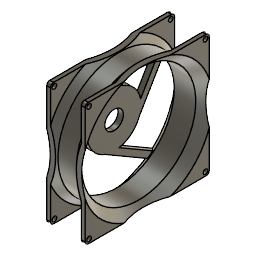
cooling_fan_pro (Autodesk Fusion 360 archive; units mm, degrees)
design "cooling fan case"
part number: 2026-04-21-22-51-45-922
Autodesk Fusion 360 part; units mm, degrees
sketch "Sketch1" plane through (0, 0, 0) normal (0, 1, 0) x (1, 0, 0)
  line L0 (0, 0) -> (7, 0)
  line L1 (7, 0) -> (12, 0) construction
  line L2 (12.5, -5.5) -> (12.5, -19.5)
  line L3 (7, 0) -> (12.5, -5.5)
  line L4 (0, -2.5) -> (5.9645, -2.5)
  line L5 (5.9645, -2.5) -> (10, -6.5355)
  line L6 (10, -6.5355) -> (10, -19.5)
  line L7 (10, -19.5) -> (12.5, -19.5)
  line L8 (0, 1) -> (0, -23) construction
  line L9 (-5.9645, -2.5) -> (-10, -6.5355)
  line L10 (-7, 0) -> (-12, 0) construction
  line L11 (0, -2.5) -> (-5.9645, -2.5)
  line L12 (0, 0) -> (-7, 0)
  line L13 (-12.5, -5.5) -> (-12.5, -19.5)
  line L14 (-10, -19.5) -> (-12.5, -19.5)
  line L15 (-7, 0) -> (-12.5, -5.5)
  line L16 (-10, -6.5355) -> (-10, -19.5)
  line L17 (0, 0) -> (0, 37) construction
  line L18 (0, 37) -> (31.2088, 37)
  dimension "d1" = 7
  dimension "d4" = 14
  dimension "d7" = 5.5
  dimension "d8" = 5.5
  dimension "d9" = 2.5
  dimension "d10" = 37
  constraint coincident L0.start L12.start
  constraint horizontal L0
  constraint horizontal L1
  constraint vertical L2
  constraint perpendicular L2 L7
  constraint perpendicular L0 L8
  constraint symmetric L0.start L8 L12.start
  constraint symmetric L0.end L8 L10.start
  constraint symmetric L2.start L8 L13.start
  constraint symmetric L1.end L8 L10.end
  constraint symmetric L2.end L8 L13.end
  constraint symmetric L4.start L8 L11.start
  constraint symmetric L4.end L8 L9.start
  constraint symmetric L5.end L8 L9.end
  constraint symmetric L6.end L8 L14.start
  constraint perpendicular L10 L17
  constraint perpendicular L17 L18
  measures "d1" distance of L0.start L0.end
  measures "d4" distance of L2.start L2.end
  measures "d7" vertical distance of L0.end L2.start
  measures "d8" horizontal distance of L0.end L2.start
  measures "d10" distance of L0.start L17.end
revolve "Revolve1" add sketch "Sketch1" angle 360 about axis through (0, 0, -37) along (1, 0, 0)
sketch "Sketch2" plane through (-12.5, 0, 0) normal (-1, 0, 0) x (0, -1, 0)
  circle A0 centre (0, -37) radius 56.5
  circle A1 centre (0, -37) radius 42.5
  circle A2 centre (0, -37) radius 56.5
  line L0 (40.2807, 2.75) -> (-40.2807, 2.75)
  line L1 (-40.2807, 2.75) -> (-40.2807, -76.75)
  line L2 (-40.2807, -76.75) -> (40.2807, -76.75)
  line L3 (40.2807, -76.75) -> (40.2807, 2.75)
  line L4 (40.2807, 2.75) -> (-40.2807, -76.75) construction
  line L5 (-40.2807, 2.75) -> (40.2807, -76.75) construction
  line L6 (72, 35) -> (-72, 35)
  line L7 (-72, 35) -> (-72, -109)
  line L8 (-72, -109) -> (72, -109)
  line L9 (72, -109) -> (72, 35)
  line L10 (72, 35) -> (-72, -109) construction
  line L11 (-72, 35) -> (72, -109) construction
  point P0 (0, -37)
  point P1 (0, -37)
  dimension "d12" = 79.5
  dimension "d13" = 144
  dimension "d14" = 144
  constraint horizontal L0
  constraint perpendicular L0 L1
  constraint parallel L0 L2
  constraint parallel L1 L3
  constraint coincident L4 P1
  constraint coincident L5 P1
  constraint coincident P1 P0
  constraint horizontal L6
  constraint perpendicular L6 L7
  constraint parallel L6 L8
  constraint parallel L7 L9
  constraint coincident L10 P1
  constraint coincident L11 P1
  measures "d12" distance of L0.end L1.end
  measures "d13" distance of L7.end L8.end
  measures "d14" distance of L6.end L7.end
extrude "Extrude1" cut sketch "Sketch2" along normal mid plane 220 contours A0 A1 A2 L3 | A0 A1 A2 L0 | A1 L3 | A0 A1 A2 L2 | A1 L0 | A1 L2 | A0 A1 A2 L1 | A1 L1 | L6 L7 L8 L9
sketch "Sketch3" plane through (-12.5, 0, 0) normal (-1, 0, 0) x (0, -1, 0)
  line L0 (40.1521, 2.75) -> (15.0395, 2.75)
  arc A0 (40.2807, -23.4459) -> (15.0395, 2.75) centre (0, -37) ccw
  line L1 (40.2807, -23.4459) -> (40.2807, 2.6196)
  arc A1 (40.2807, 2.6196) -> (40.1521, 2.75) centre (0, -37) ccw
  circle A2 centre (37.7807, 0.25) radius 1.5
  dimension "d17" = 3
  dimension "d18" = 2.5
  dimension "d19" = 2.5
  measures "d17" diameter of A2
  measures "d18" distance of L0 A2.centre
  measures "d19" distance of L1 A2.centre
extrude "Extrude2" cut sketch "Sketch3" against normal blind 95 contours A2
sketch "Sketch4" plane through (-12.5, 0, 0) normal (-1, 0, 0) x (0, -1, 0)
  circle A0 centre (37.7807, 0.25) radius 1.5
  line L0 (40.1521, 2.75) -> (15.0395, 2.75)
  arc A1 (40.2807, -23.4459) -> (15.0395, 2.75) centre (0, -37) ccw
  line L1 (40.2807, -23.4459) -> (40.2807, 2.6196)
  arc A2 (40.2807, 2.6196) -> (40.1521, 2.75) centre (0, -37) ccw
  circle A3 centre (-37.7807, 0.25) radius 1.5
  line L2 (-15.0395, 2.75) -> (-40.1521, 2.75)
  line L3 (-40.2807, 2.6196) -> (-40.2807, -23.4459)
  dimension "d22" = 3
  dimension "d23" = 2.5
  dimension "d24" = 2.5
  measures "d22" diameter of A3
  measures "d23" distance of A3.centre L2
  measures "d24" distance of A3.centre L3
extrude "Extrude3" cut sketch "Sketch4" against normal blind 65 contours A3
sketch "Sketch5" plane through (-12.5, 0, 0) normal (-1, 0, 0) x (0, -1, 0)
  line L0 (15.0395, -76.75) -> (40.1521, -76.75)
  arc A0 (40.1521, -76.75) -> (40.2807, -76.6196) centre (0, -37) ccw
  line L1 (40.2807, -76.6196) -> (40.2807, -50.5541)
  arc A1 (15.0395, -76.75) -> (40.2807, -50.5541) centre (0, -37) ccw
  circle A2 centre (37.7807, -74.25) radius 1.5
  circle A3 centre (-37.7807, -74.25) radius 1.5
  line L2 (-40.1521, -76.75) -> (-15.0395, -76.75)
  line L3 (-40.2807, -50.5541) -> (-40.2807, -76.6196)
  dimension "d27" = 3
  dimension "d28" = 2.5
  dimension "d29" = 2.5
  dimension "d30" = 3
  dimension "d31" = 2.5
  dimension "d32" = 2.5
  measures "d27" diameter of A2
  measures "d28" distance of L0 A2.centre
  measures "d29" distance of L1 A2.centre
  measures "d30" diameter of A3
  measures "d31" distance of A3.centre L2
  measures "d32" distance of A3.centre L3
extrude "Extrude4" cut sketch "Sketch5" against normal blind 30 contours A2 | A3
fillet "Fillet1" radius 2 2 edges at (-11.25, -40.1521, 2.75) (-11.25, -40.2807, 2.6196)
fillet "Fillet2" radius 2 4 edges at (11.25, -40.1521, -76.75) (11.25, -40.2807, -76.6196) (-11.25, -40.1521, -76.75) (-11.25, -40.2807, -76.6196)
fillet "Fillet3" radius 2 4 edges at (-11.25, 40.2807, -76.6196) (-11.25, 40.1521, -76.75) (11.25, 40.2807, -76.6196) (11.25, 40.1521, -76.75)
fillet "Fillet4" radius 2 4 edges at (-11.25, 40.1521, 2.75) (-11.25, 40.2807, 2.6196) (11.25, 40.1521, 2.75) (11.25, 40.2807, 2.6196)
fillet "Fillet5" radius 2 2 edges at (11.25, -40.1521, 2.75) (11.25, -40.2807, 2.6196)
sketch "Sketch6" plane through (-12.5, 0, 0) normal (-1, 0, 0) x (0, -1, 0)
  circle A0 centre (37.7807, 0.25) radius 1.5
  arc A1 (40.2807, 0.75) -> (38.2807, 2.75) centre (38.2807, 0.75) ccw
  line L0 (38.2807, 2.75) -> (15.0395, 2.75)
  arc A2 (40.2807, -23.4459) -> (15.0395, 2.75) centre (0, -37) ccw
  line L1 (40.2807, -23.4459) -> (40.2807, 0.75)
  circle A3 centre (0, -37) radius 37
  arc A4 (40.2807, -23.4459) -> (15.0395, 2.75) centre (0, -37) ccw
  line L2 (26.6601, -3.9019) -> (21.5129, -6.8969) construction
  line L3 (24.9413, -2.5881) -> (-5.8587, -20.5098)
  line L4 (28.279, -5.2738) -> (3.2929, -19.8126)
  arc A5 (-13.5541, 3.2807) -> (-39.75, -21.9605) centre (0, -37) ccw
  line L5 (-31.7262, -8.721) -> (-17.1874, -33.7071)
  line L6 (-34.4119, -12.0587) -> (-16.4902, -42.8587)
  arc A6 (-40.2807, -50.5541) -> (-15.0395, -76.75) centre (0, -37) ccw
  line L7 (-28.279, -68.7262) -> (-3.2929, -54.1874)
  line L8 (-24.9413, -71.4119) -> (5.8587, -53.4902)
  arc A7 (13.5541, -77.2807) -> (39.75, -52.0395) centre (0, -37) ccw
  line L9 (31.7262, -65.279) -> (17.1874, -40.2929)
  line L10 (34.4119, -61.9413) -> (16.4902, -31.1413)
  arc A8 (-5.8587, -20.5098) -> (-17.1874, -33.7071) centre (0, -37) ccw
  arc A9 (-16.4902, -42.8587) -> (-3.2929, -54.1874) centre (0, -37) ccw
  arc A10 (5.8587, -53.4902) -> (17.1874, -40.2929) centre (0, -37) ccw
  arc A11 (16.4902, -31.1413) -> (3.2929, -19.8126) centre (0, -37) ccw
  dimension "d49" = 360
  constraint concentric A3 A8
  constraint coincident A2 L2.start
  constraint coincident A2 L4.start
  constraint coincident A2 L3.start
  constraint coincident A3 L2.end
  constraint concentric A8 A9
  constraint concentric A9 A10
  constraint concentric A10 A11
sketch "Sketch8" plane through (-12.5, 0, 0) normal (-1, 0, 0) x (0, -1, 0)
extrude "Extrude5" add sketch "Sketch6" against normal blind 3.5 contours A2 A3 A4 L3 L4 | A3 L3 L4 L5 L6 L7 L8 L9 L10 A8 A9 A10 A11 | A3 A5 L5 L6 | A3 A7 L9 L10 | A3 A6 L7 L8
sketch "Sketch9" plane through (-9, 0, 0) normal (1, 0, 0) x (0, 1, 0)
  arc A0 (-21.6035, -4.5302) -> (-25.0811, -7.1346) centre (0, -37) ccw
  line L0 (-25.0811, -7.1346) -> (-3.2929, -19.8126)
  arc A1 (-3.2929, -19.8126) -> (-16.4902, -31.1413) centre (0, -37) ccw
  line L1 (-16.4902, -31.1413) -> (-32.4698, -58.6035)
  arc A2 (-32.4698, -58.6035) -> (-29.8654, -62.0811) centre (0, -37) ccw
  line L2 (-29.8654, -62.0811) -> (-17.1874, -40.2929)
  arc A3 (-17.1874, -40.2929) -> (-5.8587, -53.4902) centre (0, -37) ccw
  line L3 (-5.8587, -53.4902) -> (21.6035, -69.4698)
  arc A4 (21.6035, -69.4698) -> (25.0811, -66.8654) centre (0, -37) ccw
  line L4 (25.0811, -66.8654) -> (3.2929, -54.1874)
  arc A5 (3.2929, -54.1874) -> (16.4902, -42.8587) centre (0, -37) ccw
  line L5 (16.4902, -42.8587) -> (32.4698, -15.3965)
  arc A6 (32.4698, -15.3965) -> (29.8654, -11.9189) centre (0, -37) ccw
  line L6 (29.8654, -11.9189) -> (17.1874, -33.7071)
  arc A7 (17.1874, -33.7071) -> (5.8587, -20.5098) centre (0, -37) ccw
  line L7 (5.8587, -20.5098) -> (-21.6035, -4.5302)
  circle A8 centre (0, -37) radius 6
  dimension "d52" = 12
  constraint concentric A0 A8
  measures "d52" diameter of A8
extrude "Extrude6" cut sketch "Sketch9" against normal blind 15 contours A8
sketch "Sketch7" plane through (-12.5, 0, 0) normal (-1, 0, 0) x (0, -1, 0)
